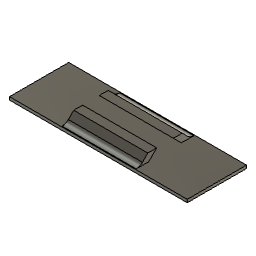
label (Autodesk Fusion 360 design; units mm, degrees)
Autodesk Fusion 360 part; units mm, degrees
sketch "Sketch1" plane through (0, 0, 0) normal (0, 0, 1) x (1, 0, 0)
  line L0 (30, -10) -> (-30, -10)
  line L1 (-30, -10) -> (-30, 10)
  line L2 (-30, 10) -> (30, 10)
  line L3 (30, 10) -> (30, -10)
  line L4 (30, -10) -> (-30, 10) construction
  line L5 (-30, -10) -> (30, 10) construction
  dimension "d1" = 60
  dimension "d2" = 20
  constraint horizontal L0
  constraint perpendicular L0 L1
  constraint parallel L0 L2
  constraint parallel L1 L3
  constraint coincident L4 origin
  constraint coincident L5 origin
  measures "d1" distance of L1.end L2.end
  measures "d2" distance of L0.end L1.end
extrude "Extrude1" add sketch "Sketch1" along normal blind 1
sketch "Sketch2" plane through (0, 0, 0) normal (1, 0, 0) x (0, 1, 0)
  line L0 (5.5, 1) -> (2.813, 3.687)
  line L1 (5.5, 1) -> (9.3, 1) construction
  line L2 (2.813, 3.687) -> (5.813, 3.687)
  line L3 (5.813, 3.687) -> (8.5, 1)
  line L4 (-5.5, 1) -> (-2.813, 3.687)
  line L5 (-5.813, 3.687) -> (-8.5, 1)
  line L6 (-2.813, 3.687) -> (-5.813, 3.687)
  line L7 (-8.5, 1) -> (-5.5, 1)
  line L8 (5.5, 1) -> (8.5, 1)
  constraint horizontal L1
  constraint horizontal L2
  constraint coincident L1 L3.end
  constraint parallel L0 L3
  constraint horizontal L7
extrude "Extrude2" add sketch "Sketch2" along normal mid plane 25
fillet "Fillet1" radius 3 2 edges at (0, -8.5, 1) (0, 8.5, 1)
